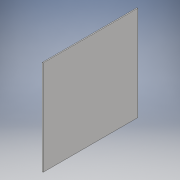
# Autodesk Inventor part: base1
Saved by Autodesk Inventor 2019 (Build 230136000, 136)
## iProperties
Created: 2020-03-02
Part Number: base1
Material: Generic
Document SubType Name: Modeling
Designer: PRAVEEN
Density: 1 g/cm^3
Appearance: Default
Author: PRAVEEN
Autodesk Inventor part; units mm, degrees
ref_plane "YZ Plane" through (0, 0, 0) normal (1, 0, 0) x (0, 1, 0)
ref_plane "XZ Plane" through (0, 0, 0) normal (0, 1, 0) x (-1, 0, 0)
ref_plane "XY Plane" through (0, 0, 0) normal (0, 0, 1) x (1, 0, 0)
sketch "Sketch1" plane through (0, 0, 0) normal (1, 0, 0) x (0, 1, 0)
  line L0 (500, 500) -> (-500, 500)
  line L1 (-500, 500) -> (-500, -500)
  line L2 (-500, -500) -> (500, -500)
  line L3 (500, -500) -> (500, 500)
  line L4 (500, 500) -> (-500, -500) construction
  line L5 (-500, 500) -> (500, -500) construction
  point P0 (0, 0)
  dimension "d0" = 1000
  dimension "d1" = 1000
  constraints: 12 end point, 2 midpoint, 2 parallel, 1 horizontal, 1 perpendicular
  measures "d0" distance of L2.end L1.end
  measures "d1" distance of L1.end L0.end
extrude "Extrusion1" add sketch "Sketch1" along normal blind 10
body "Solid1"
